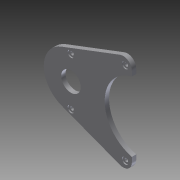
# Autodesk Inventor part: plate2
Saved by Autodesk Inventor 2012 (Build 160160000, 160)
## iProperties
Created: 2012-01-29
Part Number: plate2
Material: Default
Document SubType Name: Modeling
Designer: Antonella Wilby
Density: 1 g/cm^3
Author: Antonella Wilby
Autodesk Inventor part; units mm, degrees
ref_plane "YZ Plane" through (0, 0, 0) normal (1, 0, 0) x (0, 1, 0)
ref_plane "XZ Plane" through (0, 0, 0) normal (0, 1, 0) x (-1, 0, 0)
ref_plane "XY Plane" through (0, 0, 0) normal (0, 0, 1) x (1, 0, 0)
sketch "Sketch1" plane through (0, 0, 0) normal (0, 0, 1) x (1, 0, 0)
  line L0 (-179.705, 0) -> (89.2175, 0) projected
  line L1 (0, -106.7147) -> (0, 106.7147) projected
  circle A0 centre (0, 0) radius 50.8 construction
  arc A1 (-12.7, 50.8248) -> (-12.7, -50.8248) centre (0, 0) ccw
  line L2 (0, -55.5625) -> (0, -68.2625)
  circle A2 centre (-101.6, 0) radius 14.2875
  line L3 (-101.6, -14.2875) -> (-101.6, 14.2875) construction
  line L4 (-115.6934, 37.1008) -> (-12.7, 76.2248)
  line L5 (-115.6934, -37.1008) -> (-12.7, -76.2248)
  arc A3 (-115.6934, 37.1008) -> (-115.6934, -37.1008) centre (-101.6, 0) ccw
  line L6 (-12.7, 50.8248) -> (-12.7, 76.2248)
  line L7 (-12.7, -76.2248) -> (-12.7, -50.8248)
  dimension "d0" = 101.6
  dimension "d1" = 1.5875
  dimension "d2" = 28.575
  dimension "d4" = 101.6
  dimension "d7" = 25.4
  dimension "d8" = 25.4
  dimension "d10" = 12.7
  constraints: 12 end point, 6 point on circle, 4 centre point, 3 coincident, 3 collinear, 3 point on line, 2 tangent, 1 midpoint, 1 parallel
  measures "d0" diameter of A0
  measures "d1" radial gap between concentric circles of A1 A0
  measures "d2" diameter of A2
  measures "d4" distance between parallel lines of L1 L3
  measures "d7" radial gap between concentric circles of A3 A2
  measures "d8" distance of L6.start L4.end
  measures "d10" distance between parallel lines of L1 L6
extrude "Extrusion1" add sketch "Sketch1" along normal mid plane 6.35 contours A3 L4 L6 A1 L0 A2 | L0 A2 A1 L7 L5 A3
sketch "Sketch2" plane through (0, 0, 3.175) normal (0, 0, 1) x (1, 0, 0)
  line L0 (-12.7, 76.2248) -> (-12.7, 50.8248) projected
  line L1 (-167.005, 0) -> (13.0175, 0) projected
  point P0 (-22.225, 60.3498)
  point P1 (-22.225, -60.3498)
  dimension "d13" = 9.525
  dimension "d14" = 15.875
  constraints: 1 symmetric about line
  measures "d13" distance from line of point (-22.225, 60.35) L0
  measures "d14" vertical distance of L0.start point (-22.225, 60.35)
hole "Hole1" at (-22.225, 60.3498, 3.175) at (-22.225, -60.3498, 3.175) direction (0, 0, -1) diameter 5.1054 end through all counterbore diameter 9.779 counterbore depth 1.5875 clearance for "Flat Head Machine Screw (82)" size "#10" standard "Ansi Unified Screw Threads"
fillet "Fillet1" radius 12.7 1 edges at (-12.7, 76.2248, 0)
fillet "Fillet1" radius 12.7 1 edges at (-12.7, -76.2248, 0)
sketch "Sketch3" plane through (0, 0, 3.175) normal (0, 0, 1) x (1, 0, 0)
  arc A0 (-115.6934, 37.1008) -> (-115.6934, -37.1008) centre (-101.6, 0) ccw projected
  line L0 (-169.545, 0) -> (28.2575, 0) projected
  point P0 (-101.6, 34.925)
  point P1 (-101.6, -34.925)
  dimension "d24" = 34.925
  constraints: 1 symmetric about line, 1 vertical alignment
  measures "d24" distance from line of point (-101.6, 34.925) L0
hole "Hole2" at (-101.6, 34.925, 3.175) at (-101.6, -34.925, 3.175) direction (0, 0, -1) diameter 5.1054 end through all counterbore diameter 9.779 counterbore depth 1.5875 clearance for "Flat Head Machine Screw (82)" size "#10" standard "Ansi Unified Screw Threads"
body "Solid1"
